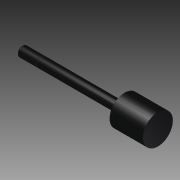
# Autodesk Inventor part: C-040.5-DP0_rod
Saved by Autodesk Inventor 2011 SP1 (Build 150282100, 282)
## iProperties
Created: 2015-01-23
Part Number: C-040.5-DP0_rod
Catalog Web Link: www.cadenas.de
Description: Standard Air Cylinder_rod-Original Line - Standard Air Cylinders
Vendor: BIMBA
Document SubType Name: Modeling
Designer: psAdmin
Manufacturer: BIMBA
Mass: 8.31564 g
Surface Area: 31.9434 cm^2
Volume: 8.31564 cm^3
Density: 1 g/cm^3
Category: PARTsolutions
Company: BIMBA
Title: C-040.5-DP0_rod
Author: Cadenas PARTsolutions
Comments: Original Line - Standard Air Cylinders
PSOL_IDENT_0: {$CADENAS_DATA\23d-libs\bimba\bimba\bimba_imperial\bimba_full_line\original_line_cylinders\standard_
PSOL_IDENT_1: air_cylinders\rod.prj},284 {VTYP=3D},{NB=C-040.5-DP0_rod},{LINA=C-040.5-DP0_rod},{NN=Standard Air Cy
PSOL_IDENT_2: linder_rod},{DATE=08.09.2014 05:04:05},{GEOMDATE=08.09.2014 05:04:01},{VERSION=},{LINEID=50},{LINESU
PSOL_IDENT_3: BID=-1},{WBVAR=STROKE,ACTING,MNT,DER,NR,BM,CO,M,EE,EEL,K,Q,Y,F,G,T,B,H,SER,SR,NT,W,E,HL,ST,STP,PRC,P
PSOL_IDENT_4: B,COLOR1}  {NB=C-040.5-DP0_rod},{LINA=C-040.5-DP0_rod},{KT=DUMMY},{PN=C-040.5-DP},{DASH=-},{BORE=0.7
PSOL_IDENT_5: 5000000},{BOREPN=04},{STROKE=0.500},{STROKEALG=[0.001:50/0.001]},{STROKE1=0.500},{ACTING=D},{ACTINGA
PSOL_IDENT_6: LG= '' , 'Single Acting' , 'R' , 'Reverse Single Acting' , 'D' , 'Double Acting' },{ACTINGPN=D},{MNT=
PSOL_IDENT_7: P},{MNTALG= '' , 'Front Nose Mounting' , 'P' , 'Rear Pivot Mounting' , 'XP' , 'Double End or Pivot M
PSOL_IDENT_8: ounting' , 'X' , 'Double End Mounting' , 'BF' , 'Front Block Mounting' , 'BR' , 'Rear Block Mounting
PSOL_IDENT_9: for Vertical Positioning' , 'BFT' , 'Front Block Trunnion Mounting' , 'BRT' , 'Rear Block Trunnion
PSOL_IDENT_10: Mounting' },{TYPE=C-},{MNTPN=P},{DER=},{DERALG= '' , 'N/A' },{NR=},{NRALG= '' , 'N/A' },{NRPN=},{BM=
PSOL_IDENT_11: },{BMALG= '' , 'N/A' },{BMPN=},{CO=},{COALG= '' , 'N/A' },{M=},{MALG= '', 'Without Magnet', 'M', 'Wi
PSOL_IDENT_12: th Magnet' },{EE=},{EEL=0},{EEMAX=12},{EEALG= '', 'Without Extra Extension', 'EE', 'With Extra Exten
PSOL_IDENT_13: sion' },{EELALG=0},{EEPN=},{EEPN1=0.000},{K=},{KALG= '', 'Standard' , 'K' , 'Ports Rotated 90deg' },
PSOL_IDENT_14: {KPN=},{Q=},{QALG= '' , 'Without Side Ported Rear Head' , 'Q' , 'With Side Ported Rear Head' },{QPN=
PSOL_IDENT_15: },{Y=},{YALG= '' , 'Without Pivot Bushing' , 'Y' , 'With Pivot Bushing' },{YPN=},{F=},{FALG= '', 'St
PSOL_IDENT_16: andard', 'F', 'Molycoated Body' },{FPN=},{G=},{GPN=},{T=},{TALG= '' , 'Standard' , 'N' , 'Low Temper
PSOL_IDENT_17: ature' , 'V' , 'High Temperature' },{NPN=},{VPN=},{B=},{BALG= '', 'Without Bumper' , 'B' , 'With Bum
PSOL_IDENT_18: per' },{BPN=},{H=},{HALG= '', 'N/A' },{HPN=},{SER=},{SERALG= '' , 'Without Spring Extend/Return' , '
PSOL_IDENT_19: JS' , 'With Spring Return' , 'JR' , 'With Spring Extend' },{SR=C},{SRALG= 'C' , 'Carbon Steel Rod' ,
PSOL_IDENT_20: 'SR' , '303 Stainless Steel Rod' , '' , '303 Stainless Steel Rod1' },{SRPN=C},{SRCON=1},{NT=},{NTPN=
PSOL_IDENT_21: },{W=},{WALG= '' , 'Without Wiper' , 'W' , 'With Wiper' },{WPN=},{E=},{EALG= '' , 'Without Special L
PSOL_IDENT_22: ube and Seals' , 'E' , 'With Special Lube and Seals' },{EPN=},{HL=},{HLALG= '' , 'Wihout Low Pressur
PSOL_IDENT_23: e Hydraulic' , 'HL' , 'With Low Pressure Hydraulic' },{ST=},{STALG= '' , 'Without Switch Track' , 'T'
PSOL_IDENT_24: , 'With Switch Track' },{STP=},{STPALG= '' , 'N/A' },{STPN=},{PRC=},{PRCALG= '' , 'Without Piston R
PSOL_IDENT_25: od Clevis' , 'D-166-1' , 'With Piston Rod Clevis' },{PRCPN=},{PB=},{PBALG= '' , 'Without Pivot Brack
PSOL_IDENT_26: et' , 'D-167' , 'With Pivot Bracket' },{PBPN=},{TLEN=1.7555},{TEXT=0.133333},{SPACE=0.07619},{FRAC=3
PSOL_IDENT_27: .7500},{RGCON=},{RGDACCON=R},{RHCON=P},{RHCONON=1},{RHACCON=},{FNUTCON=0},{RNUTCON=0},{FNUTPN=},{RNU
PSOL_IDENT_28: TPN=},{FNUTTRANS=0.0000},{RNUTTRANS=0.0000},{VHOLECON=0},{A1=1.5940},{A1N=0.8750},{A1P=1.5940},{A1B=
PSOL_IDENT_29: 1.5940},{A4=0.2525},{A4N=0.3130},{A4P=0.2525},{A5=0.0300},{A1H=1.594},{A1NH=0.5310},{A1PH=1.5940},{A
PSOL_IDENT_30: 1BH=1.0940},{A1SH=1.2190},{A2H=0.2190},{A2NH=0.2190},{LENGTH=3.7500},{LENGTH1=3.7500},{LENGTH2=3.810
PSOL_IDENT_31: 0},{MUL=0.5000},{MUL11=0.5000},{MUL22=1.3450},{MUL33=0.8450},{MUL2=0.5000},{MUL211=0.5000},{MUL222=2
PSOL_IDENT_32: .6900},{MUL233=1.6900},{SSS=0.5000},{RGLEN=1.3715},{RHLEN=1.1230},{SSS1=1.0000},{A13=1.3120},{THDLEN
PSOL_IDENT_33: 1=0.5000},{THD1=0.2500},{TAB=UNF},{THDLEN=0.5000},{THD=0.2500},{OD=0.7615},{RODL=3.4380},{PL=0.8440}
PSOL_IDENT_34: ,{RODDIA=0.2500},{HEX=0.2500},{RODTRANS=0.0000},{G1=0.1250},{ON=0},{G5=0.6250},{DERLEN=2.5940},{THOL
PSOL_IDENT_35: E=0.0000},{WF=0.2200},{BADD=0.0000},{MADD=0.0000},{NVADD=0.000},{JRADD=0.00000},{COLOR=0.00,0.00,0.0
PSOL_IDENT_36: 0,0.00},{GROOVE=1},{HOL=0},{D7=0.2520},{H1=1.1175},{D1=0.8625},{D1RH=0.8625},{D1P=0.8325},{D1B=0.862
PSOL_IDENT_37: 5},{D1N=0.8050},{D1NRH=0.8050},{D1BRH=0.8325},{D1PRH=0.8625},{BOZO=0},{HADD=0.000},{COLOR1=0},{DEFL=
PSOL_IDENT_38: 0.0000},{HEXL=0.0000},{SSADD=0.0000},{WFL=0.0000},{MOVE=0.0000},{PRCL2=0.50000},{PRCB=0.16000},{PRCT
PSOL_IDENT_39: RANS=0.16000}
SUPPLIER: BIMBA
ARTICLENO: C-040.5-DP0_rod
BOMINFO: C-040.5-DP0_rod
CREATOR: CADENAS GmbH
Autodesk Inventor part; units mm, degrees
ref_plane "YZ Plane" through (0, 0, 0) normal (1, 0, 0) x (0, 1, 0)
ref_plane "XZ Plane" through (0, 0, 0) normal (0, 1, 0) x (-1, 0, 0)
ref_plane "XY Plane" through (0, 0, 0) normal (0, 0, 1) x (1, 0, 0)
sketch "Sketch_1" plane through (0, 0, 0) normal (0, 0, 1) x (1, 0, 0)
  line L0 (74.6252, 0) -> (0, 0)
  line L1 (0, 0) -> (0, 3.175)
  line L2 (0, 3.175) -> (53.1876, 3.175)
  line L3 (53.1876, 3.175) -> (53.1876, 9.6203)
  line L4 (53.1876, 9.6203) -> (74.6252, 9.6203)
  line L5 (74.6252, 9.6203) -> (74.6252, 0)
  line L6 (74.6252, 0) -> (0, 0)
  constraints: 14 end point
revolve "Revolution1" add sketch "Sketch_1" angle 360 about axis through (74.6252, 0, 0) along (1, 0, 0)
sketch "Sketch_3" plane through (0, 0, 0) normal (0, 0, 1) x (1, 0, 0)
  line L0 (0, 0) -> (-12.7, 0)
  line L1 (-12.7, 0) -> (-12.7, 2.634)
  line L2 (-12.7, 2.634) -> (-12.159, 3.175)
  line L3 (-12.159, 3.175) -> (0, 3.175)
  line L4 (0, 3.175) -> (0, 0)
  line L5 (0, 0) -> (-12.7, 0)
  constraints: 12 end point
revolve "Revolution2" add sketch "Sketch_3" angle 360 about axis through (0, 0, 0) along (1, 0, 0)
sketch "Sketch_30" plane through (0, 0, 0) normal (0, 0, 1) x (1, 0, 0)
  line L0 (0, 0) -> (-0.254, 0)
  line L1 (-0.254, 3.429) -> (-0.254, 2.921)
  line L2 (-0.254, 2.921) -> (0, 2.921)
  line L3 (0, 2.921) -> (0, 3.429)
  line L4 (0, 3.429) -> (-0.254, 3.429)
  constraints: 10 end point
revolve "Revolution3" cut sketch "Sketch_30" angle 360 about axis through (0, 0, 0) along (1, 0, 0)
ref_plane "dia1_XY" through (0, 3.175, 0) normal (1, 0, 0) x (0, 0, -1)
ref_plane "dia1_YZ" through (0, 3.175, 0) normal (0, 0, -1) x (0, 1, 0)
ref_plane "dia1_ZX" through (0, 3.175, 0) normal (0, 1, 0) x (1, 0, 0)
ref_plane "dia12_XY" through (0, 0, 10.9537) normal (1, 0, 0) x (0, 0, -1)
ref_plane "dia12_YZ" through (0, 0, 10.9537) normal (0, 0, -1) x (0, 1, 0)
ref_plane "dia12_ZX" through (0, 0, 10.9537) normal (0, 1, 0) x (1, 0, 0)
ref_plane "dia2_XY" through (0, -3.175, 0) normal (1, 0, 0) x (0, 0, -1)
ref_plane "dia2_YZ" through (0, -3.175, 0) normal (0, 0, -1) x (0, 1, 0)
ref_plane "dia2_ZX" through (0, -3.175, 0) normal (0, 1, 0) x (1, 0, 0)
ref_plane "dia22_XY" through (0, 0, -10.9537) normal (1, 0, 0) x (0, 0, -1)
ref_plane "dia22_YZ" through (0, 0, -10.9537) normal (0, 0, -1) x (0, 1, 0)
ref_plane "dia22_ZX" through (0, 0, -10.9537) normal (0, 1, 0) x (1, 0, 0)
ref_plane "rl1_XY" through (-12.7, 0, 0) normal (1, 0, 0) x (0, 0, -1)
ref_plane "rl1_YZ" through (-12.7, 0, 0) normal (0, 0, -1) x (0, 1, 0)
ref_plane "rl1_ZX" through (-12.7, 0, 0) normal (0, 1, 0) x (1, 0, 0)
ref_plane "rl2_XY" through (0, 0, 0) normal (1, 0, 0) x (0, 0, -1)
ref_plane "rl2_YZ" through (0, 0, 0) normal (0, 0, -1) x (0, 1, 0)
ref_plane "rl2_ZX" through (0, 0, 0) normal (0, 1, 0) x (1, 0, 0)
ref_plane "rod_cp_XY" through (0, 0, 0) normal (1, 0, 0) x (0, 0, -1)
ref_plane "rod_cp_YZ" through (0, 0, 0) normal (0, 0, -1) x (0, 1, 0)
ref_plane "rod_cp_ZX" through (0, 0, 0) normal (0, 1, 0) x (1, 0, 0)
ref_plane "thd1_XY" through (-12.7, 3.175, 0) normal (1, 0, 0) x (0, 0, -1)
ref_plane "thd1_YZ" through (-12.7, 3.175, 0) normal (0, 0, -1) x (0, 1, 0)
ref_plane "thd1_ZX" through (-12.7, 3.175, 0) normal (0, 1, 0) x (1, 0, 0)
ref_plane "thd2_XY" through (-12.7, -3.175, 0) normal (1, 0, 0) x (0, 0, -1)
ref_plane "thd2_YZ" through (-12.7, -3.175, 0) normal (0, 0, -1) x (0, 1, 0)
ref_plane "thd2_ZX" through (-12.7, -3.175, 0) normal (0, 1, 0) x (1, 0, 0)
ref_plane "to_rod_clevis_XY" through (-16.764, 0, 0) normal (1, 0, 0) x (0, 0, -1)
ref_plane "to_rod_clevis_YZ" through (-16.764, 0, 0) normal (0, 0, -1) x (0, 1, 0)
ref_plane "to_rod_clevis_ZX" through (-16.764, 0, 0) normal (0, 1, 0) x (1, 0, 0)
body "Solid1"
